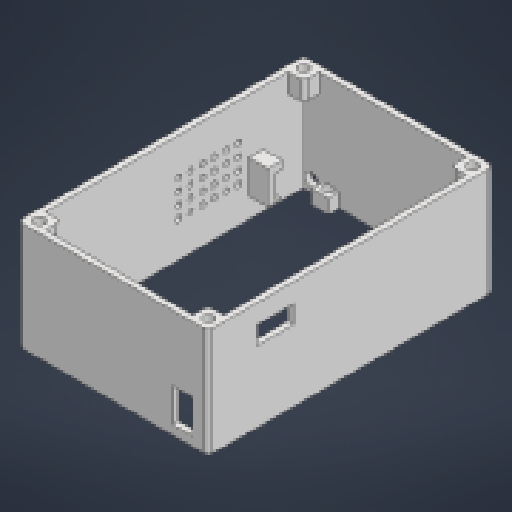
# Autodesk Inventor part: PCB_Housing_03_V4
Saved by Autodesk Inventor 2026.2 (Build 302298000, 298)
## iProperties
Created: 2026-03-15
Part Number: PCB_Housing_03_V4
Material: Generic
Document SubType Name: Modeling
Designer: vckot
Density: 1 g/cm^3
Appearance: Default
Author: vckot
Autodesk Inventor part; units mm, degrees
ref_plane "YZ Plane" through (0, 0, 0) normal (1, 0, 0) x (0, 1, 0)
ref_plane "XZ Plane" through (0, 0, 0) normal (0, 1, 0) x (-1, 0, 0)
ref_plane "XY Plane" through (0, 0, 0) normal (0, 0, 1) x (1, 0, 0)
sketch "Sketch2" plane through (0, 0, 0) normal (0, 1, 0) x (1, 0, 0)
  line L0 (40, -60) -> (40, 60)
  line L1 (40, 60) -> (-40, 60)
  line L2 (-40, 60) -> (-40, -60)
  line L3 (-40, -60) -> (40, -60)
  line L4 (-37.5, -57.5) -> (-37.5, 57.5)
  line L5 (-37.5, 57.5) -> (37.5, 57.5)
  line L6 (37.5, 57.5) -> (37.5, -57.5)
  line L7 (37.5, -57.5) -> (-37.5, -57.5)
  line L8 (32.5, -37.5) -> (37.5, -37.5)
  line L9 (32.5, -37.5) -> (32.5, -40)
  line L10 (32.5, -40) -> (37.5, -40)
  point P0 (0, 0)
  point P1 (40, 0)
  point P2 (0, 60)
  point P3 (0, 0)
  dimension "d4" = 2.5
  dimension "d7" = 120
  dimension "d8" = 80
  dimension "d9" = 20
  dimension "d10" = 5
  dimension "d11" = 2.5
  constraints: 22 end point, 4 perpendicular, 2 midpoint, 2 point on line, 1 coincident, 1 horizontal, 1 horizontal alignment, 1 vertical, 1 vertical alignment, 3 other
  measures "d4" distance between parallel lines of L2 L4
  measures "d7" distance of L0.start L0.end
  measures "d8" distance of L0.end L1.end
  measures "d9" distance between parallel lines of L7 L8
  measures "d10" distance of L8.start L8.end
  measures "d11" distance of L8.start L9.end
extrude "Extrusion2" add sketch "Sketch2" along normal blind 45.5
extrude "Extrusion3" add sketch "Sketch2" along normal blind 2.5 contours L10 L9 L8 L6
sketch "Sketch3" plane through (-37.5, 0, 57.5) normal (1, 0, 0) x (0, 0, -1)
  line L0 (95.08, 8.5) -> (95.08, 22.5)
  line L1 (115, 0) -> (115, 45.5) projected
  line L2 (95.08, 8.5) -> (92.08, 8.5)
  line L3 (92.08, 8.5) -> (92.08, 22.5)
  line L4 (117.5, 0) -> (-2.5, 0) projected
  line L5 (95.08, 22.5) -> (92.08, 22.5)
  point P0 (57.5, 0)
  dimension "d14" = 19.92
  dimension "d15" = 3
  dimension "d16" = 8.5
  dimension "d17" = 14
  constraints: 8 end point, 2 horizontal, 1 perpendicular, 1 vertical
  measures "d14" distance between parallel lines of L1 L0
  measures "d15" distance between parallel lines of L0 L3
  measures "d16" distance between parallel lines of L4 L2
  measures "d17" distance between parallel lines of L2 L5
extrude "Extrusion4" add sketch "Sketch3" along normal blind 8
sketch "Sketch4" plane through (-37.5, 8.5, -37.58) normal (0, 0, -1) x (-1, 0, 0)
  line L0 (-8, 0) -> (-8, 14) projected
  line L1 (-8, 0) -> (0, 0)
  line L2 (0, 0) -> (0, 1)
  line L3 (0, 1) -> (-8, 1)
  line L4 (-8, 1) -> (-8, 0)
  line L5 (0, 14) -> (0, 0) projected
  line L6 (0, 0) -> (-8, 0) projected
  point P0 (-37.5, -8.5)
  point P1 (-8, 1)
  dimension "d20" = 1
  constraints: 8 end point, 2 parallel, 1 collinear, 1 horizontal, 1 perpendicular
  measures "d20" distance between parallel lines of L6 L3
extrude "Extrusion5" add sketch "Sketch4" along normal blind 2
sketch "Sketch5" plane through (0, 0, 0) normal (0, -1, 0) x (1, 0, 0)
  line L0 (-40, 60) -> (40, 60) projected
  line L1 (-40, 60) -> (-33, 60)
  line L2 (-33, 60) -> (-33, 53)
  line L3 (-33, 53) -> (-40, 53)
  line L4 (-40, 53) -> (-40, 60)
  line L5 (40, 60) -> (40, -60) projected
  line L6 (40, 60) -> (33, 60)
  line L7 (33, 60) -> (33, 53)
  line L8 (33, 53) -> (40, 53)
  line L9 (40, 53) -> (40, 60)
  line L10 (40, -60) -> (-40, -60) projected
  line L11 (-29.5, -60) -> (-22.5, -60)
  line L12 (-22.5, -60) -> (-22.5, -53)
  line L13 (-22.5, -53) -> (-29.5, -53)
  line L14 (-29.5, -53) -> (-29.5, -60)
  line L15 (-29.5, -34.58) -> (-29.5, -39.58) projected
  point P0 (0, 0)
  dimension "d23" = 7
  dimension "d24" = 7
  dimension "d25" = 7
  dimension "d26" = 7
  dimension "d27" = 7
  dimension "d28" = 7
  dimension "d29" = 0
  constraints: 24 end point, 6 parallel, 3 horizontal, 3 perpendicular, 1 point on line
  measures "d23" distance of L2.end L3.end
  measures "d24" distance of L1.end L2.end
  measures "d25" distance of L8.end L7.end
  measures "d26" distance of L7.end L6.end
  measures "d27" distance of L13.end L12.end
  measures "d28" distance of L12.end L11.end
  measures "d29" distance between parallel lines of L15 L14
extrude "Extrusion6" add sketch "Sketch5" against normal blind 6
sketch "Sketch6" plane through (0, 0, 0) normal (0, -1, 0) x (1, 0, 0)
  line L0 (-37.5, 53) -> (-33, 53) projected
  line L1 (-33, 53) -> (-33, 57.5) projected
  line L2 (33, 53) -> (37.5, 53) projected
  line L3 (33, 57.5) -> (33, 53) projected
  line L4 (40, -60) -> (-40, -60) projected
  line L5 (-22.5, -57.5) -> (-22.5, -53) projected
  point P0 (0, 0)
  point P1 (-26, -56.5)
  point P2 (-36.5, 56.5)
  point P3 (36.5, 56.5)
  point P4 (35.25, 53)
  dimension "d32" = 3.5
  dimension "d33" = 3.5
  dimension "d34" = 3.5
  dimension "d35" = 3.5
  dimension "d36" = 3.5
  dimension "d37" = 3.5
  constraints: 1 midpoint
  measures "d32" distance from line of L0 point (-36.5, 56.5)
  measures "d33" distance from line of L1 point (-36.5, 56.5)
  measures "d34" vertical distance of point (35.25, 53) point (36.5, 56.5)
  measures "d35" distance from line of L3 point (36.5, 56.5)
  measures "d36" distance from line of L4 point (-26, -56.5)
  measures "d37" distance from line of L5 point (-26, -56.5)
hole "Hole1" at (-26, 0, -56.5) at (-36.5, 0, 56.5) at (36.5, 0, 56.5) direction (0, 1, 0) diameter 4.5 depth 6 tip angle 118
sketch "Sketch7" plane through (0, 45.5, 0) normal (0, 1, 0) x (1, 0, 0)
  line L0 (-40, 60) -> (-40, -60) projected
  line L1 (-40, 60) -> (-31, 60)
  line L2 (-31, 60) -> (-31, 51)
  line L3 (-31, 51) -> (-40, 51)
  line L4 (-40, 51) -> (-40, 60)
  line L5 (-40, -60) -> (40, -60) projected
  line L6 (40, -60) -> (31, -60)
  line L7 (31, -60) -> (31, -51)
  line L8 (31, -51) -> (40, -51)
  line L9 (40, -51) -> (40, -60)
  line L10 (-40, -60) -> (-31, -60)
  line L11 (-31, -60) -> (-31, -51)
  line L12 (-31, -51) -> (-40, -51)
  line L13 (-40, -51) -> (-40, -60)
  line L14 (40, 60) -> (-40, 60) projected
  line L15 (40, 60) -> (31, 60)
  line L16 (31, 60) -> (31, 51)
  line L17 (31, 51) -> (40, 51)
  line L18 (40, 51) -> (40, 60)
  point P0 (0, 0)
  point P1 (-35.5, 55.5)
  point P2 (-31, 55.5)
  point P3 (-35.5, 51)
  point P4 (-35.5, -55.5)
  point P5 (35.5, 55.5)
  point P6 (-31, -55.5)
  point P7 (35.5, 51)
  point P8 (35.5, -55.5)
  dimension "d45" = 9
  dimension "d46" = 9
  dimension "d47" = 9
  dimension "d48" = 9
  dimension "d63" = 9
  dimension "d64" = 9
  dimension "d65" = 9
  dimension "d66" = 9
  constraints: 32 end point, 8 parallel, 4 horizontal, 4 horizontal alignment, 4 midpoint, 4 perpendicular, 4 vertical alignment
  measures "d45" distance of L2.end L3.end
  measures "d46" distance of L1.end L2.end
  measures "d47" distance of L7.end L8.end
  measures "d48" distance of L6.end L7.end
  measures "d63" distance of L12.end L11.end
  measures "d64" distance of L11.end L10.end
  measures "d65" distance of L17.end L16.end
  measures "d66" distance of L16.end L15.end
extrude "Extrusion7" add sketch "Sketch7" against normal blind 8
hole "Hole2" at (-35.5, 45.5, -55.5) at (35.5, 45.5, -55.5) at (-35.5, 45.5, 55.5) at (35.5, 45.5, 55.5) direction (0, -1, 0) diameter 4.5 depth 8 tip angle 118
fillet "Fillet1" radius 2 4 edges at (-40, 22.75, 60) (40, 22.75, 60) (-40, 22.75, -60) (40, 22.75, -60)
sketch "Sketch8" plane through (-37.5, 0, 53) normal (1, 0, 0) x (0, 0, -1)
  line L0 (90.58, 22.5) -> (90.58, 9.5) projected
  line L1 (90.58, 19.5) -> (93.58, 19.5)
  line L2 (93.58, 19.5) -> (93.58, 22.5)
  line L3 (93.58, 22.5) -> (90.58, 22.5)
  line L4 (87.58, 22.5) -> (90.58, 22.5) projected
  point P0 (53, 0)
  dimension "d59" = 3
  dimension "d60" = 3
  constraints: 6 end point, 2 perpendicular, 1 collinear, 1 point on line
  measures "d59" distance between parallel lines of L0 L2
  measures "d60" distance between parallel lines of L3 L1
extrude "Extrusion8" add sketch "Sketch8" along normal up to surface (8 mm away)
sketch "Sketch9" plane through (40, 0, 58) normal (1, 0, 0) x (0, 0, -1)
  line L0 (24.82, 30.9115) -> (23.72, 30.9115) projected
  line L1 (22.28, 30.9115) -> (21.18, 30.9115) projected
  line L2 (30.78, 30.9115) -> (29.68, 30.9115) projected
  line L3 (33.32, 30.9115) -> (32.22, 30.9115) projected
  line L4 (33.32, 30.9115) -> (27.32, 30.9115)
  line L5 (27.32, 30.9115) -> (27.32, 24.9115)
  line L6 (27.32, 24.9115) -> (33.32, 24.9115)
  line L7 (33.32, 24.9115) -> (33.32, 30.9115)
  line L8 (24.97, 30.9115) -> (18.97, 30.9115)
  line L9 (18.97, 30.9115) -> (18.97, 24.9115)
  line L10 (18.97, 24.9115) -> (24.97, 24.9115)
  line L11 (24.97, 24.9115) -> (24.97, 30.9115)
  line L12 (18.97, 30.9115) -> (33.32, 30.9115)
  line L13 (33.32, 30.9115) -> (33.32, 36.9115)
  line L14 (33.32, 36.9115) -> (18.97, 36.9115)
  line L15 (18.97, 36.9115) -> (18.97, 30.9115)
  point P0 (58, 0)
  dimension "d67" = 6
  dimension "d68" = 6
  dimension "d69" = 6
  dimension "d70" = 6
  dimension "d71" = 2.35
  dimension "d101" = 6
  dimension "d102" = 14.35
  constraints: 24 end point, 6 parallel, 3 horizontal, 3 perpendicular, 1 point on line
  measures "d67" distance of L6.end L5.end
  measures "d68" distance of L5.end L4.end
  measures "d69" distance of L10.end L9.end
  measures "d70" distance of L9.end L8.end
  measures "d71" distance between parallel lines of L5 L11
  measures "d101" distance of L13.end L12.end
  measures "d102" distance of L13.end L14.end
extrude "Extrusion9" cut sketch "Sketch9" against normal up to surface (2.5 mm away) contours L0 L8 L1 L15 L14 L13 L3 L4 L2 L12
sketch "Sketch13" plane through (-37.5, 0, 53) normal (1, 0, 0) x (0, 0, -1)
  line L0 (78.06, 7.2265) -> (78.06, 2.2265) projected
  line L1 (0, 0) -> (110.5, 0) projected
  line L2 (78.06, 10) -> (82.06, 10)
  line L3 (82.06, 10) -> (82.06, 0)
  line L4 (82.06, 0) -> (78.06, 0)
  line L5 (78.06, 0) -> (78.06, 10)
  point P0 (53, 0)
  dimension "d111" = 4
  dimension "d112" = 10
  constraints: 8 end point, 2 parallel, 2 point on line, 1 horizontal, 1 perpendicular
  measures "d111" distance of L3.end L4.end
  measures "d112" distance of L2.end L3.end
extrude "Extrusion13" add sketch "Sketch13" along normal blind 7.5
thicken "Thicken2" operation add thickness 0.5 both sides no extend neighbours yes toward (0, 0, -1) faces at (39.1667, 32.9115, 24.68) (39.1667, 30.9115, 34.2467) (39.1667, 36.9115, 29.4633) (39.1667, 34.9115, 39.03)
sketch "Sketch10" plane through (38, 0, -60) normal (0, 0, -1) x (-1, 0, 0)
  circle A0 centre (72.3, 5) radius 2.509
  line L0 (78, 0) -> (78, 45.5) projected
  line L1 (0, 0) -> (76, 0) projected
  point P0 (38, 0)
  dimension "d80" = 5.018
  dimension "d109" = 5.7
  dimension "d110" = 5
  constraints: 1 centre point
  measures "d80" diameter of A0
  measures "d109" distance from line of L0 A0.centre
  measures "d110" distance from line of L1 A0.centre
extrude "Extrusion10" cut sketch "Sketch10" against normal up to surface (34.94 mm away)
fillet "Fillet4" radius 2 2 edges at (-30, 10, -27.06) (-30, 0, -27.06)
sketch "Sketch11" plane through (-40, 0, -58) normal (-1, 0, 0) x (0, 0, 1)
  circle A0 centre (28, 30) radius 1.25
  line L0 (-2, 45.5) -> (-2, 0) projected
  line L1 (0, 0) -> (116, 0) projected
  circle A1 centre (28, 25) radius 1.25
  circle A2 centre (28, 20) radius 1.25
  circle A3 centre (28, 15) radius 1.25
  circle A4 centre (33, 30) radius 1.25
  circle A5 centre (33, 25) radius 1.25
  circle A6 centre (33, 20) radius 1.25
  circle A7 centre (33, 15) radius 1.25
  circle A8 centre (38, 30) radius 1.25
  circle A9 centre (38, 25) radius 1.25
  circle A10 centre (38, 20) radius 1.25
  circle A11 centre (38, 15) radius 1.25
  circle A12 centre (43, 30) radius 1.25
  circle A13 centre (43, 25) radius 1.25
  circle A14 centre (43, 20) radius 1.25
  circle A15 centre (43, 15) radius 1.25
  circle A16 centre (48, 30) radius 1.25
  circle A17 centre (48, 25) radius 1.25
  circle A18 centre (48, 20) radius 1.25
  circle A19 centre (48, 15) radius 1.25
  circle A20 centre (53, 30) radius 1.25
  circle A21 centre (53, 25) radius 1.25
  circle A22 centre (53, 20) radius 1.25
  circle A23 centre (53, 15) radius 1.25
  point P0 (58, 0)
  dimension "d83" = 2.5
  dimension "d84" = 30
  dimension "d85" = 30
  dimension "d88" = 5
  dimension "d91" = 5
  constraints: 24 centre point, 1 horizontal, 1 vertical, 46 other
  measures "d83" diameter of A0
  measures "d84" distance from line of L0 A0.centre
  measures "d85" distance from line of L1 A0.centre
  measures "d88" distance of A0.centre A1.centre
  measures "d91" distance of A0.centre A4.centre
extrude "Extrusion11" cut sketch "Sketch11" against normal up to surface (2.5 mm away)
sketch "Sketch12" plane through (-38, 0, 60) normal (0, 0, 1) x (1, 0, 0)
  line L0 (53.5, 1) -> (53.5, 21) projected
  line L1 (74.5, 1) -> (53.5, 1) projected
  line L2 (74.5, 21) -> (74.5, 1) projected
  line L3 (53.5, 21) -> (74.5, 21) projected
  line L4 (64, 21) -> (64, 1)
  line L5 (64, 17) -> (70.5, 17)
  line L6 (70.5, 17) -> (70.5, 5)
  line L7 (70.5, 5) -> (64, 5)
  line L8 (64, 5) -> (64, 17)
  line L9 (71.5, 18) -> (63, 18)
  line L10 (63, 18) -> (63, 4)
  line L11 (63, 4) -> (71.5, 4)
  line L12 (71.5, 4) -> (71.5, 18)
  point P0 (38, 0)
  point P1 (70.5, 11)
  point P2 (74.5, 11)
  dimension "d104" = 12
  dimension "d105" = 6.5
  dimension "d106" = 1
  constraints: 18 end point, 4 midpoint, 4 parallel, 2 perpendicular, 1 horizontal, 1 horizontal alignment, 1 point on line, 3 other
  measures "d104" distance of L5.end L6.end
  measures "d105" distance of L5.start L5.end
  measures "d106" distance between parallel lines of L5 L9
extrude "Extrusion12" cut sketch "Sketch12" against normal up to surface (2.5 mm away) contours L11 L10 L9 L4 | L4 L7 L6 L5 L9 L12 L11 | L4 L5 L6 L7
fillet "Fillet2" radius 2 4 edges at (-31, 41.5, -51) (31, 41.5, -51) (31, 41.5, 51) (-31, 41.5, 51)
fillet "Fillet3" radius 1 4 edges at (25, 18, 58.75) (25, 4, 58.75) (33.5, 18, 58.75) (33.5, 4, 58.75)
sketch "Sketch14" plane through (-37.5, 0, 53) normal (1, 0, 0) x (0, 0, -1)
  line L0 (78.06, 2.491) -> (78.06, 7.509) projected
  line L1 (56.125, 8.175) -> (56.125, 1.825)
  line L2 (56.125, 8.175) -> (49.875, 8.175)
  line L3 (49.875, 8.175) -> (49.875, 1.825)
  line L4 (49.875, 1.825) -> (56.125, 1.825)
  line L5 (56.125, 1.825) -> (56.125, 8.175)
  line L6 (111, 45.5) -> (-5, 45.5) projected
  line L7 (48.875, 9.175) -> (57.125, 9.175)
  line L8 (57.125, 9.175) -> (57.125, 0.825)
  line L9 (57.125, 0.825) -> (48.875, 0.825)
  line L10 (48.875, 0.825) -> (48.875, 9.175)
  line L11 (51.375, 8.175) -> (51.375, 9.175)
  line L12 (54.625, 8.175) -> (54.625, 9.175)
  line L13 (56.125, 6.675) -> (57.125, 6.675)
  line L14 (56.125, 3.325) -> (57.125, 3.325)
  line L15 (54.625, 1.825) -> (54.625, 0.825)
  line L16 (51.375, 1.825) -> (51.375, 0.825)
  line L17 (49.875, 3.325) -> (48.875, 3.325)
  line L18 (49.875, 6.675) -> (48.875, 6.675)
  point P0 (56.125, 5)
  point P1 (78.06, 5)
  point P2 (53, 8.175)
  point P3 (53, 45.5)
  point P4 (49.375, 6.675)
  point P5 (51.375, 8.675)
  point P6 (56.125, 6.675)
  point P7 (56.125, 3.325)
  dimension "d116" = 6.35
  dimension "d117" = 6.25
  dimension "d118" = 6.35
  dimension "d119" = 1
  dimension "d120" = 2.5
  dimension "d121" = 2.5
  dimension "d122" = 2.5
  dimension "d123" = 2.5
  constraints: 34 end point, 22 point on line, 7 perpendicular, 6 midpoint, 4 parallel, 1 collinear, 1 horizontal, 1 horizontal alignment, 1 vertical, 1 vertical alignment, 3 other
  measures "d116" distance of L1.start L1.end
  measures "d117" distance of L4.end L3.end
  measures "d118" distance between parallel lines of L4 L2
  measures "d119" distance between parallel lines of L2 L7
  measures "d120" distance from line of point (49.375, 6.675) L7
  measures "d121" distance from line of L10 point (51.375, 8.675)
  measures "d122" distance between parallel lines of L8 L12
  measures "d123" distance between parallel lines of L9 L17
extrude "Extrusion14" add sketch "Sketch14" along normal blind 1 contours L2 L12 L7 L8 L13 L1 | L14 L8 L9 L15 L4 L1 | L2 L3 L18 L10 L7 L11 | L16 L9 L10 L17 L3 L4
thicken "Thicken5" operation add thickness 3 both sides no extend neighbours yes toward (0, -1, 0) faces at (-39.1667, 45.5, 17)
body "Solid1"
